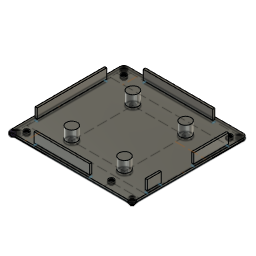
bottom_cover (Autodesk Fusion 360 design; units mm, degrees)
Autodesk Fusion 360 part; units mm, degrees
sketch "Sketch5" plane through (0, 0, 0) normal (0, 0, 1) x (1, 0, 0)
  line L0 (1.5, 0) -> (84.5, 0) construction
  line L1 (86, 1.5) -> (86, 78.5) construction
  line L2 (84.5, 80) -> (1.5, 80) construction
  line L3 (0, 78.5) -> (0, 1.5) construction
  arc A0 (1.5, 80) -> (0, 78.5) centre (1.5, 78.5) ccw construction
  arc A1 (86, 78.5) -> (84.5, 80) centre (84.5, 78.5) ccw construction
  arc A2 (84.5, 0) -> (86, 1.5) centre (84.5, 1.5) ccw construction
  arc A3 (0, 1.5) -> (1.5, 0) centre (1.5, 1.5) ccw construction
  circle A4 centre (81, 75) radius 1.85
  circle A5 centre (66, 5) radius 1.85
  circle A6 centre (5, 5) radius 1.85
  circle A7 centre (5, 75) radius 1.85
  line L4 (66, 5) -> (66, 0) construction
  line L5 (5, 5) -> (5, 0) construction
  line L6 (5, 5) -> (0, 5) construction
  line L7 (5, 75) -> (5, 80) construction
  line L8 (5, 75) -> (0, 75) construction
  line L9 (81, 75) -> (86, 75) construction
  line L10 (81, 75) -> (81, 80) construction
  line L11 (66, 5) -> (86, 5) construction
  line L12 (15.5875, 79.9) -> (65.5875, 79.9)
  line L13 (65.5875, 79.9) -> (65.5875, 78.4)
  line L14 (65.5875, 78.4) -> (15.5875, 78.4)
  line L15 (15.5875, 78.4) -> (15.5875, 79.9)
  line L16 (15.3114, 1.6) -> (55.3114, 1.6)
  line L17 (55.3114, 1.6) -> (55.3114, 0.1)
  line L18 (55.3114, 0.1) -> (15.3114, 0.1)
  line L19 (15.3114, 0.1) -> (15.3114, 1.6)
  line L20 (84.4, 69.451) -> (85.9, 69.451)
  line L21 (85.9, 69.451) -> (85.9, 44.451)
  line L22 (85.9, 44.451) -> (84.4, 44.451)
  line L23 (84.4, 44.451) -> (84.4, 69.451)
  line L24 (0.1, 66.068) -> (1.6, 66.068)
  line L25 (1.6, 66.068) -> (1.6, 16.068)
  line L26 (1.6, 16.068) -> (0.1, 16.068)
  line L27 (0.1, 16.068) -> (0.1, 66.068)
  line L28 (0.5, 70) -> (85.5, 70) construction
  line L29 (85.5, 70) -> (85.5, 10) construction
  line L30 (85.5, 10) -> (0.5, 10) construction
  line L31 (0.5, 10) -> (0.5, 70) construction
  line L32 (9.3353, 80) -> (9.3353, 70) construction
  line L33 (9.3353, 10) -> (9.3353, 0) construction
  line L34 (85.5, 36.8145) -> (86, 36.8145) construction
  line L35 (0.5, 33.1865) -> (0, 33.1865) construction
  line L36 (26, 60.5) -> (64, 60.5) construction
  line L37 (64, 60.5) -> (64, 16.5) construction
  line L38 (64, 16.5) -> (26, 16.5) construction
  line L39 (26, 16.5) -> (26, 60.5) construction
  line L40 (64, 53.3314) -> (85.5, 53.3314) construction
  line L41 (-1.5, 78.5) -> (-1.5, 1.5)
  arc A8 (-1.5, 1.5) -> (1.5, -1.5) centre (1.5, 1.5) ccw
  line L42 (1.5, -1.5) -> (84.5, -1.5)
  arc A9 (84.5, -1.5) -> (87.5, 1.5) centre (84.5, 1.5) ccw
  line L43 (87.5, 1.5) -> (87.5, 78.5)
  arc A10 (87.5, 78.5) -> (84.5, 81.5) centre (84.5, 78.5) ccw
  line L44 (84.5, 81.5) -> (1.5, 81.5)
  arc A11 (1.5, 81.5) -> (-1.5, 78.5) centre (1.5, 78.5) ccw
  circle A12 centre (26, 60.5) radius 4
  circle A13 centre (64, 60.5) radius 4
  circle A14 centre (64, 16.5) radius 4
  circle A15 centre (26, 16.5) radius 4
  line L45 (84.4, 21.0236) -> (85.9, 21.0236)
  line L46 (85.9, 21.0236) -> (85.9, 11.0236)
  line L47 (85.9, 11.0236) -> (84.4, 11.0236)
  line L48 (84.4, 11.0236) -> (84.4, 21.0236)
  point P0 (86, 0)
  point P1 (0, 80)
  dimension "d11" = 86
  dimension "d12" = 80
  dimension "d13" = 1.5
  dimension "d14" = 1.5
  dimension "d15" = 1.5
  dimension "d16" = 1.5
  dimension "d17" = 3.7
  dimension "d18" = 5
  dimension "d19" = 20
  dimension "d20" = 50
  dimension "d21" = 1.5
  dimension "d22" = 40
  dimension "d23" = 1.5
  dimension "d24" = 1.5
  dimension "d25" = 25
  dimension "d26" = 1.5
  dimension "d27" = 50
  dimension "d28" = 0.1
  dimension "d29" = 0.1
  dimension "d30" = 0.1
  dimension "d31" = 0.1
  dimension "d32" = 85
  dimension "d33" = 60
  dimension "d34" = 38
  dimension "d35" = 44
  dimension "d36" = 21.5
  dimension "d37" = 6.5
  dimension "d38" = 1.5
  dimension "d39" = 8
  dimension "d42" = 1.5
  dimension "d43" = 10
  dimension "d44" = 0.1
  constraint horizontal L0
  constraint vertical L1
  constraint horizontal L2
  constraint vertical L3
  constraint coincident P1 L2
  constraint coincident P1 L3
  constraint tangent L2 A0
  constraint tangent L3 A0
  constraint tangent L1 A1
  constraint tangent L2 A1
  constraint coincident P0 L0
  constraint coincident P0 L1
  constraint tangent L0 A2
  constraint tangent L1 A2
  constraint coincident origin L0
  constraint coincident origin L3
  constraint tangent L0 A3
  constraint tangent L3 A3
  constraint equal A4 A7
  constraint equal A4 A6
  constraint equal A4 A5
  constraint coincident A5.centre L4.start
  constraint coincident L0 L4.end
  constraint perpendicular L0 L4
  constraint coincident A6.centre L5.start
  constraint coincident L0 L5.end
  constraint perpendicular L0 L5
  constraint coincident L3 L6.end
  constraint perpendicular L3 L6
  constraint coincident A7.centre L7.start
  constraint coincident L2 L7.end
  constraint perpendicular L2 L7
  constraint coincident L3 L8.end
  constraint perpendicular L3 L8
  constraint coincident A4.centre L9.start
  constraint coincident L1 L9.end
  constraint perpendicular L1 L9
  constraint coincident L2 L10.end
  constraint perpendicular L2 L10
  constraint equal L9 L10
  constraint equal L7 L10
  constraint equal L7 L8
  constraint equal L5 L6
  constraint equal L6 L8
  constraint equal L4 L5
  constraint coincident L1 L11.end
  constraint perpendicular L1 L11
  constraint horizontal L12
  constraint vertical L13
  constraint horizontal L14
  constraint vertical L15
  constraint horizontal L16
  constraint vertical L17
  constraint horizontal L18
  constraint vertical L19
  constraint horizontal L20
  constraint vertical L21
  constraint horizontal L22
  constraint vertical L23
  constraint horizontal L24
  constraint vertical L25
  constraint horizontal L26
  constraint vertical L27
  constraint horizontal L28
  constraint vertical L29
  constraint horizontal L30
  constraint vertical L31
  constraint coincident L2 L32.start
  constraint coincident L28 L32.end
  constraint perpendicular L28 L32
  constraint coincident L30 L33.start
  constraint coincident L0 L33.end
  constraint perpendicular L0 L33
  constraint coincident L29 L34.start
  constraint coincident L1 L34.end
  constraint perpendicular L1 L34
  constraint coincident L31 L35.start
  constraint coincident L3 L35.end
  constraint perpendicular L3 L35
  constraint equal L34 L35
  constraint equal L32 L33
  constraint horizontal L36
  constraint vertical L37
  constraint horizontal L38
  constraint vertical L39
  constraint coincident L37 L40.start
  constraint coincident L29 L40.end
  constraint perpendicular L29 L40
  constraint coincident L36.start L39.end
  constraint coincident L36.end L37.start
  constraint coincident L37.end L38.start
  constraint coincident L38.end L39.start
  constraint equal A12 A13
  constraint equal A14 A15
  constraint equal A12 A15
  constraint horizontal L45
  constraint vertical L46
  constraint horizontal L47
  constraint vertical L48
  measures "d11" distance of origin P0
  measures "d12" distance of origin P1
  measures "d13" radius of A0
  measures "d14" radius of A1
  measures "d15" radius of A2
  measures "d16" radius of A3
  measures "d17" diameter of A4
  measures "d18" distance of A4.centre L10.end
  measures "d19" distance of A5.centre L11.end
  measures "d20" distance of L12.start L12.end
  measures "d21" distance of L12.start L14.end
  measures "d22" distance of L16.start L16.end
  measures "d23" distance of L16.start L18.end
  measures "d24" distance of L20.start L20.end
  measures "d25" distance of L20.start L22.end
  measures "d26" distance of L24.start L24.end
  measures "d27" distance of L24.start L26.end
  measures "d28" distance of L2 L12
  measures "d29" distance of L1 L21
  measures "d30" distance of L3 L27
  measures "d31" distance of L0 L18
  measures "d32" distance of L28.start L28.end
  measures "d33" distance of L28.start L30.end
  measures "d34" distance of L36.start L36.end
  measures "d35" distance of L36.start L38.end
  measures "d36" distance of L40.start L40.end
  measures "d37" distance of L30 L38
  measures "d39" diameter of A13
  measures "d42" distance of L45.start L45.end
  measures "d43" distance of L45.start L47.end
  measures "d44" distance of L1 L46
extrude "Extrude3" add sketch "Sketch5" along normal blind 8.5 contours L12 L13 L14 L15 | L16 L17 L18 L19 | L20 L21 L22 L23 | L24 L25 L26 L27 | L45 L46 L47 L48 makes body 1 at (85.9, 17.6902, 2.8333) makes body 2 at (84.4, 52.7844, 2.8333) makes body 3 at (28.6448, 1.6, 2.8333) makes body 4 at (48.9208, 78.4, 2.8333) makes body 5 at (1.6, 49.4013, 2.8333)
extrude "Extrude2" add sketch "Sketch5" along normal blind 1.5 separate body makes body 6
extrude "Extrude4" add sketch "Sketch5" along normal blind 9.5 contours A12 | A13 | A14 | A15 bodies 6
